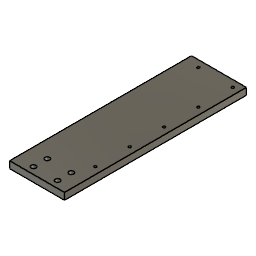
cover rolls mount right (Autodesk Fusion 360 design; units mm, degrees)
Autodesk Fusion 360 part; units mm, degrees
note: some values were not read from the file. Set by a fixed rule: which face or edge a step refers to.
sketch "Szkic1" plane through (0, 0, 0) normal (0, 0, 1) x (1, 0, 0)
  line L0 (-35, -15) -> (35, -15)
  line L1 (35, -15) -> (35, 0)
  line L2 (35, 0) -> (35, 40)
  line L3 (35, 40) -> (-35, 40)
  line L4 (-35, 40) -> (-35, -15)
  circle A0 centre (-20, 15) radius 2
  circle A1 centre (-20, -5) radius 2
  circle A2 centre (15, -5) radius 2
  circle A3 centre (15, 15) radius 2
  line L5 (-35, 0) -> (-35, 250)
  line L6 (35, 0) -> (35, 250)
  line L7 (-35, 250) -> (35, 250)
  line L8 (-35, -15) -> (-17, -15)
  line L9 (-17, 250) -> (-35, 250)
  line L10 (-35, 250) -> (-35, -15)
  line L11 (35, -15) -> (35, 250)
  circle A4 centre (25, 240) radius 1.75
  circle A5 centre (-25, 240) radius 1.75
  circle A6 centre (25, 190) radius 1.75
  circle A7 centre (25, 140) radius 1.75
  circle A8 centre (25, 90) radius 1.75
  circle A9 centre (25, 40) radius 1.75
  dimension "d1" = 250
  dimension "d2" = 250
  dimension "d3" = 3.5
  dimension "d4" = 3.5
  dimension "d5" = 3.5
  dimension "d6" = 3.5
  dimension "d7" = 3.5
  dimension "d8" = 3.5
  constraint coincident L4 L5.start
  constraint perpendicular L3 L5
  constraint perpendicular L3 L6
  constraint perpendicular L5 L7
  constraint parallel L8 L9
  constraint perpendicular L4 L8
  constraint perpendicular L7 L11
  constraint coincident L3 A9.centre
  measures "d1" distance of L5.start L5.end
  measures "d2" distance of L1.end L6.end
  measures "d3" diameter of A4
  measures "d4" diameter of A5
  measures "d5" diameter of A6
  measures "d6" diameter of A7
  measures "d7" diameter of A8
  measures "d8" diameter of A9
extrude "Wyciągnięcie proste1" add sketch "Szkic1" along normal blind 10 contours L0 L1 L2 L3 L4 L5 L6 L8 L10 L11 A9 | L3 L5 L6 L7 L9 L10 L11 A9
extrude "Wyciągnięcie proste2" add 3 faces at (-35, -5, 3.3333) (-35, 110, 6.6667) (-35, 26.6667, 3.3333) along direction (-1, 0, 0) blind 10
sketch "Szkic2" plane through (0, 0, 10) normal (0, 0, 1) x (-1, 0, 0)
  circle A0 centre (-25, -240) radius 1.75
  circle A1 centre (20, 5) radius 2
  circle A2 centre (20, -15) radius 2
  circle A3 centre (-25, -190) radius 1.75
  circle A4 centre (25, -240) radius 1.75
  circle A5 centre (-15, 5) radius 2
  circle A6 centre (-25, -40) radius 1.75
  circle A7 centre (-25, -90) radius 1.75
  circle A8 centre (-25, -140) radius 1.75
  circle A9 centre (-15, -15) radius 2
  line L0 (-35, -250) -> (45, -250)
  line L1 (45, -250) -> (45, 15)
  line L2 (45, 15) -> (-35, 15)
  line L3 (-35, 15) -> (-35, -250)
  circle A10 centre (-15, -15) radius 3.5
  circle A11 centre (-15, 5) radius 3.5
  circle A12 centre (20, -15) radius 3.5
  circle A13 centre (20, 5) radius 3.5
  dimension "d13" = 7
  dimension "d14" = 7
  dimension "d15" = 7
  dimension "d16" = 7
  constraint concentric A9 A10
  constraint concentric A5 A11
  constraint concentric A2 A12
  constraint concentric A1 A13
  measures "d13" diameter of A10
  measures "d14" diameter of A11
  measures "d15" diameter of A12
  measures "d16" diameter of A13
extrude "Wyciągnięcie proste3" cut sketch "Szkic2" against normal blind 5 contours A10 | A11 | A12 | A13
sketch "Szkic3" plane through (0, 0, 0) normal (0, 0, -1) x (1, 0, 0)
  circle A0 centre (25, -240) radius 1.75
  circle A1 centre (-20, 5) radius 2
  circle A2 centre (-20, -15) radius 2
  circle A3 centre (25, -190) radius 1.75
  circle A4 centre (-25, -240) radius 1.75
  circle A5 centre (15, 5) radius 2
  circle A6 centre (25, -40) radius 1.75
  circle A7 centre (25, -90) radius 1.75
  circle A8 centre (25, -140) radius 1.75
  circle A9 centre (15, -15) radius 2
  line L0 (-45, -250) -> (35, -250)
  line L1 (35, -250) -> (35, 15)
  line L2 (35, 15) -> (-45, 15)
  line L3 (-45, 15) -> (-45, -250)
  circle A10 centre (25, -40) radius 3.5
  circle A11 centre (25, -90) radius 3.5
  circle A12 centre (25, -140) radius 3.5
  circle A13 centre (25, -190) radius 3.5
  circle A14 centre (25, -240) radius 3.5
  circle A15 centre (-25, -240) radius 3.5
  dimension "d19" = 7
  dimension "d20" = 7
  dimension "d21" = 7
  dimension "d22" = 7
  dimension "d23" = 7
  dimension "d24" = 7
  constraint concentric A6 A10
  constraint concentric A7 A11
  constraint concentric A8 A12
  constraint concentric A3 A13
  constraint concentric A0 A14
  constraint concentric A4 A15
  measures "d19" diameter of A10
  measures "d20" diameter of A11
  measures "d21" diameter of A12
  measures "d22" diameter of A13
  measures "d23" diameter of A14
  measures "d24" diameter of A15
extrude "Wyciągnięcie proste4" cut sketch "Szkic3" against normal blind 5 contours A10 | A11 | A12 | A13 | A14 | A15
